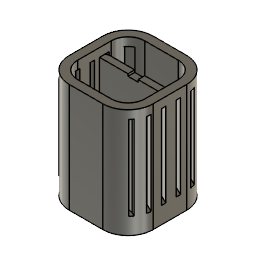
Sensor Casing (Autodesk Fusion 360 design; units mm, degrees)
Autodesk Fusion 360 part; units mm, degrees
sketch "Sketch1" plane through (0, 0, 0) normal (0, 0, 1) x (1, 0, 0)
  line L0 (10, 0) -> (30, 0)
  line L1 (40, 10) -> (40, 30)
  line L2 (30, 40) -> (10, 40)
  line L3 (0, 30) -> (0, 10)
  line L4 (0, 25) -> (40, 25) construction
  line L5 (0, 27) -> (40, 27)
  line L6 (0, 23) -> (40, 23)
  line L7 (10, -5) -> (30, -5)
  line L8 (45, 10) -> (45, 30)
  line L9 (30, 45) -> (10, 45)
  line L10 (-5, 30) -> (-5, 10)
  line L11 (9.4326, 16.3) -> (30.5674, 16.3)
  line L12 (30.5674, 2) -> (9.4326, 2)
  line L13 (20, 40) -> (20, 0) construction
  line L14 (20, 16.3) -> (20, 2) construction
  line L15 (37.5, 9.15) -> (2.5, 9.15) construction
  line L16 (8.5, 16.3) -> (8.5, 2) construction
  line L17 (31.5, 16.3) -> (31.5, 2) construction
  line L18 (7.9005, 15.5856) -> (3.5789, 10.4356)
  line L19 (7.9005, 2.7144) -> (3.5789, 7.8644)
  line L20 (32.0995, 2.7144) -> (36.4211, 7.8644)
  line L21 (32.0995, 15.5856) -> (36.4211, 10.4356)
  arc A0 (9.4326, 16.3) -> (7.9005, 15.5856) centre (9.4326, 14.3) ccw
  arc A1 (32.0995, 15.5856) -> (30.5674, 16.3) centre (30.5674, 14.3) ccw
  arc A2 (36.4211, 7.8644) -> (36.4211, 10.4356) centre (34.8891, 9.15) ccw
  arc A3 (30.5674, 2) -> (32.0995, 2.7144) centre (30.5674, 4) ccw
  arc A4 (7.9005, 2.7144) -> (9.4326, 2) centre (9.4326, 4) ccw
  arc A5 (3.5789, 10.4356) -> (3.5789, 7.8644) centre (5.1109, 9.15) ccw
  arc A6 (10, 40) -> (0, 30) centre (10, 30) ccw
  arc A7 (40, 30) -> (30, 40) centre (30, 30) ccw
  arc A8 (30, 0) -> (40, 10) centre (30, 10) ccw
  arc A9 (0, 10) -> (10, 0) centre (10, 10) ccw
  arc A10 (10, 45) -> (-5, 30) centre (10, 30) ccw
  arc A11 (45, 30) -> (30, 45) centre (30, 30) ccw
  arc A12 (30, -5) -> (45, 10) centre (30, 10) ccw
  arc A13 (-5, 10) -> (10, -5) centre (10, 10) ccw
  point P0 (40, 0)
  point P1 (0, 40)
  point P2 (-5, -5)
  point P3 (45, -5)
  point P4 (-5, 45)
  dimension "d1" = 40
  dimension "d2" = 40
  dimension "d3" = 25
  dimension "d4" = 2
  dimension "d5" = 2
  dimension "d6" = 50
  dimension "d7" = 50
  dimension "d10" = 2
  dimension "d13" = 6
  dimension "d14" = 6
  dimension "d15" = 14.3
  dimension "d16" = 35
  dimension "d17" = 2
  dimension "d18" = 2
  dimension "d41" = 10
  dimension "d42" = 15
  dimension "d43" = 15
  dimension "d44" = 15
  dimension "d45" = 15
  constraint horizontal L0
  constraint vertical L1
  constraint horizontal L2
  constraint vertical L3
  constraint coincident L3 L4.start
  constraint coincident L1 L4.end
  constraint perpendicular L1 L4
  constraint coincident L3 L5.start
  constraint coincident L1 L5.end
  constraint perpendicular L1 L5
  constraint coincident L3 L6.start
  constraint coincident L1 L6.end
  constraint perpendicular L1 L6
  constraint horizontal L7
  constraint vertical L8
  constraint horizontal L9
  constraint vertical L10
  constraint horizontal L11
  constraint horizontal L12
  constraint collinear L13 L14
  constraint perpendicular L12 L16
  constraint perpendicular L12 L17
  constraint coincident L11 L14.start
  constraint coincident L12 L14.end
  constraint coincident L11 L16.start
  constraint coincident L16.start L18
  constraint tangent L11 A0
  constraint tangent L18 A0
  constraint coincident L17.start L21
  constraint coincident L11 L17.start
  constraint tangent L21 A1
  constraint tangent L11 A1
  constraint equal A0 A1
  constraint coincident L15.start L21
  constraint coincident L15.start L20
  constraint tangent L21 A2
  constraint tangent L20 A2
  constraint equal A0 A2
  constraint coincident L17.end L20
  constraint coincident L12 L17.end
  constraint tangent L20 A3
  constraint tangent L12 A3
  constraint equal A0 A3
  constraint coincident L12 L16.end
  constraint coincident L16.end L19
  constraint tangent L12 A4
  constraint tangent L19 A4
  constraint equal A0 A4
  constraint coincident L15.end L19
  constraint coincident L15.end L18
  constraint tangent L19 A5
  constraint tangent L18 A5
  constraint coincident L2 L13.start
  constraint coincident P1 L2
  constraint coincident P1 L3
  constraint tangent L2 A6
  constraint tangent L3 A6
  constraint tangent L1 A7
  constraint tangent L2 A7
  constraint equal A6 A7
  constraint coincident L0 L13.end
  constraint coincident P0 L0
  constraint coincident P0 L1
  constraint tangent L0 A8
  constraint tangent L1 A8
  constraint equal A6 A8
  constraint coincident origin L0
  constraint coincident origin L3
  constraint tangent L0 A9
  constraint tangent L3 A9
  constraint equal A6 A9
  constraint coincident P4 L9
  constraint coincident P4 L10
  constraint tangent L9 A10
  constraint tangent L10 A10
  constraint tangent L8 A11
  constraint tangent L9 A11
  constraint coincident P3 L7
  constraint coincident P3 L8
  constraint tangent L7 A12
  constraint tangent L8 A12
  constraint coincident P2 L7
  constraint coincident P2 L10
  constraint tangent L7 A13
  constraint tangent L10 A13
  measures "d1" distance of origin P0
  measures "d2" distance of origin P1
  measures "d3" distance of L0 L4
  measures "d4" distance of L4 L5
  measures "d5" distance of L4 L6
  measures "d6" distance of P2 P3
  measures "d7" distance of P2 P4
  measures "d10" distance of L0 L12
  measures "d13" distance of L15.start L17
  measures "d14" distance of L15.end L16
  measures "d15" distance of L11 L12
  measures "d16" distance of L15.start L15.end
  measures "d17" radius of A0
  measures "d18" radius of A5
  measures "d41" radius of A6
  measures "d42" radius of A10
  measures "d43" radius of A11
  measures "d44" radius of A12
  measures "d45" radius of A13
extrude "Extrude1" add sketch "Sketch1" along normal blind 60 contours L1 L3 L5 L6 | L7 L8 L9 L10 A10 A11 A12 A13
extrude "Extrude2" add sketch "Sketch1" against normal blind 5 contours L0 L1 L3 L6 A8 A9 | L1 L3 L5 L6 | L1 L2 L3 L5 A6 A7 | L7 L8 L9 L10 A10 A11 A12 A13
sketch "Sketch2" plane through (0, 0, 60) normal (0, 0, 1) x (-1, 0, 0)
  line L0 (-30, 0) -> (-10, 0)
  line L1 (0, -10) -> (0, -23)
  line L2 (-40, -23) -> (-40, -10)
  line L3 (-10, -40) -> (-30, -40)
  line L4 (5, -30) -> (5, -10)
  line L5 (-10, 5) -> (-30, 5)
  line L6 (-45, -10) -> (-45, -30)
  line L7 (-30, -45) -> (-10, -45)
  line L8 (-10, -40) -> (5, -32.5)
  line L9 (5, -35) -> (0, -37.5)
  line L10 (0, -37.5) -> (-10, -40)
  line L11 (5, -35) -> (5, -32.5)
  arc A0 (-40, -30) -> (-30, -40) centre (-30, -30) ccw
  arc A1 (-30, 0) -> (-40, -10) centre (-30, -10) ccw
  arc A2 (0, -10) -> (-10, 0) centre (-10, -10) ccw
  arc A3 (-10, -40) -> (0, -30) centre (-10, -30) ccw
  arc A4 (5, -10) -> (-10, 5) centre (-10, -10) ccw
  arc A5 (-30, 5) -> (-45, -10) centre (-30, -10) ccw
  arc A6 (-45, -30) -> (-30, -45) centre (-30, -30) ccw
  arc A7 (-10, -45) -> (5, -30) centre (-10, -30) ccw
  line L12 (0, -23) -> (-40, -23)
  line L13 (-40, -30) -> (-40, -27)
  line L14 (-40, -27) -> (0, -27)
  line L15 (0, -27) -> (0, -30)
  constraint coincident L3.start L8.start
  constraint coincident L4 L8.end
  constraint coincident L4 L9.start
  constraint parallel L8 L9
extrude "Extrude3" cut sketch "Sketch2" along normal blind -55 and the other way blind 5 contours L8 L10 A3 | L8 L9 L10 A3 A7 | L8 L9 L11 A7
pattern_linear "R-Pattern1" count 5 spacing 8.75 along (0, -1, 0) of "Extrude3"
ref_plane "WorkPlane1" through (20, 28.5, 30) normal (-1, 0, 0) x (0, -1, 0)
mirror "Mirror1" about plane through (20, 28.5, 30) normal (-1, 0, 0) of "Extrude3"
mirror "Mirror2" about plane through (20, 28.5, 30) normal (-1, 0, 0) of "R-Pattern1"
sketch "Sketch3" plane through (0, 0, 60) normal (0, 0, 1) x (-1, 0, 0)
  line L0 (-30, 0) -> (-10, 0)
  line L1 (0, -10) -> (0, -23)
  line L2 (-40, -23) -> (-40, -10)
  line L3 (-10, -40) -> (-30, -40)
  line L4 (5, -30) -> (5, -10)
  line L5 (-10, 5) -> (-30, 5)
  line L6 (-45, -10) -> (-45, -30)
  line L7 (-30, -45) -> (-10, -45)
  line L8 (0, -27) -> (-40, -27)
  line L9 (-40, -27) -> (-40, -23)
  line L10 (-40, -23) -> (0, -23)
  line L11 (0, -23) -> (0, -27)
  line L12 (-17, -27) -> (-23, -27)
  line L13 (-23, -27) -> (-23, -23)
  line L14 (-23, -23) -> (-17, -23)
  line L15 (-17, -23) -> (-17, -27)
  line L16 (-20, -27) -> (-20, -23) construction
  line L17 (-20, -27) -> (-20, -23) construction
  arc A0 (-40, -30) -> (-30, -40) centre (-30, -30) ccw
  arc A1 (-30, 0) -> (-40, -10) centre (-30, -10) ccw
  arc A2 (0, -10) -> (-10, 0) centre (-10, -10) ccw
  arc A3 (-10, -40) -> (0, -30) centre (-10, -30) ccw
  arc A4 (5, -10) -> (-10, 5) centre (-10, -10) ccw
  arc A5 (-30, 5) -> (-45, -10) centre (-30, -10) ccw
  arc A6 (-45, -30) -> (-30, -45) centre (-30, -30) ccw
  arc A7 (-10, -45) -> (5, -30) centre (-10, -30) ccw
  line L18 (0, -23) -> (-40, -23)
  line L19 (-40, -30) -> (-40, -27)
  line L20 (-40, -27) -> (0, -27)
  line L21 (0, -27) -> (0, -30)
  dimension "d36" = 6
  constraint horizontal L8
  constraint vertical L9
  constraint horizontal L10
  constraint vertical L11
  constraint coincident L2.start L9.end
  constraint horizontal L12
  constraint vertical L13
  constraint horizontal L14
  constraint vertical L15
  constraint coincident L8 L12.start
  constraint midpoint L8 L16.start
  constraint midpoint L10 L16.end
  constraint midpoint L12 L16.start
  constraint midpoint L14 L16.end
  constraint collinear L16 L17
  measures "d36" distance of L12.start L12.end
extrude "Extrude4" cut sketch "Sketch3" against normal blind 5 contours L8 L9 L10 L13 L18 L20 | L8 L10 L11 L15 L18 L20
extrude "Extrude5" cut 1 faces at (19, 25.6667, 60) along direction (0, 0, -1) blind 6.3
